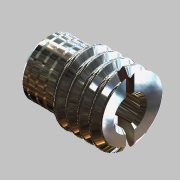
# Autodesk Inventor part: YTP-AP-E04-R1.0
Saved by Autodesk Inventor 2020.4 (Build 244396010, 396A)
## iProperties
Created: 2021-08-28
Part Number: YTP-AP-E04-R1.0
Material: Edelstahl
Document SubType Name: Modeling
Designer: Uwe Wieser
Mass: 0.28749 g
Surface Area: 1.23286 cm^2
Volume: 0.0359362 cm^3
Density: 8 g/cm^3
Appearance: Chrom - poliert
Project: Airbrush
Description: Dichtungsschraube
Werkstoff: 1.4301
Author: Uwe Wieser
Autodesk Inventor part; units mm, degrees
sketch "Skizze1" plane through (0, 0, 0) normal (0, 0, 1) x (1, 0, 0)
  line L0 (0, -0.4978) -> (0, 2.9869) projected
  line L1 (-3.8336, 0) -> (4.9014, 0) projected
  line L2 (-2.5857, 0.8) -> (-2.5857, 1.647)
  line L3 (2.4143, 2) -> (2.4143, 0.8)
  line L4 (-0.9352, 2) -> (-0.8754, 2) construction
  line L5 (-1.0857, 1.8366) -> (-0.8106, 1.8366) construction
  line L6 (-0.5857, 2) -> (-0.5857, 2.4891) construction
  line L7 (-1.5857, 2) -> (-1.5857, 2.1811) construction
  line L8 (-2.0857, 2) -> (-2.0857, 2.2584) construction
  line L9 (-2.0857, 1.4574) -> (-2.0167, 1.647)
  line L10 (-2.0857, 1.4574) -> (-2.1547, 1.647)
  line L11 (-0.5857, 2) -> (2.4143, 2)
  line L12 (-1.5166, 1.647) -> (-1.5876, 1.647) construction
  line L13 (-1.5166, 1.647) -> (-1.1547, 1.647)
  line L14 (-2.5857, 1.647) -> (-2.1547, 1.647)
  line L15 (-2.0167, 1.647) -> (-1.6548, 1.647)
  line L16 (-2.5857, 0.8) -> (2.4143, 0.8)
  line L17 (-1.1547, 1.647) -> (-1.0857, 1.4574)
  line L18 (-1.6548, 1.647) -> (-1.5856, 1.4574)
  line L19 (-1.5856, 1.4574) -> (-1.5166, 1.647)
  line L20 (-1.0857, 1.4574) -> (-1.0167, 1.647)
  line L21 (-1.0857, 1.4574) -> (-0.884, 1.4574) construction
  line L22 (-1.0167, 1.647) -> (-0.5857, 1.647)
  line L23 (-0.5857, 1.647) -> (-0.5857, 2)
  line L24 (3.2727, 1.57) -> (3.6536, 1.57) construction
  line L25 (2.4143, 1.8644) -> (3.0263, 1.8644) construction
  line L26 (2.4143, 1.8644) -> (3.0252, 1.8644) construction
  line L27 (3.3514, 1.57) -> (3.1921, 1.57) construction
  point P0 (0, 0)
  dimension "d7" = 2
  dimension "d8" = 0.5
  dimension "d9" = 0.5
  dimension "d10" = 0.5
  dimension "d16" = 1.6
  dimension "d19" = 3.294
  dimension "d21" = 70
  dimension "d22" = 4
  dimension "d42" = 5
  dimension "d43" = 110
  dimension "d44" = 110
  dimension "d45" = 0.1383
  dimension "d46" = 0.138
  dimension "d47" = 0.138
  dimension "d100" = 0.353
  constraints: 52 end point, 8 horizontal, 7 perpendicular, 3 horizontal alignment, 3 point on line, 3 symmetric about line, 3 vertical, 2 equal length
  measures "d7" distance from line of L6 L2.end
  measures "d8" distance from line of L6 L5.start
  measures "d9" distance from line of L5.start L7
  measures "d10" distance between parallel lines of L8 L7
  measures "d16" diameter of L16 L1
  measures "d19" diameter of L13 L1
  measures "d21" angle of L21 L20
  measures "d22" diameter of L11 L1
  measures "d42" distance of L3.end L2.start
  measures "d43" angle of L14 L10
  measures "d44" angle of L17 L13
  measures "d45" distance of L12.start L15.end
  measures "d46" distance of L9.end L10.end
  measures "d47" distance of L20.end L13.end
  measures "d100" distance of L22.end L6.start
revolve "Umdrehung1" add sketch "Skizze1" angle 360 about axis through (-10, 0, 0) along (1, 0, 0)
ref_plane "Arbeitsebene1" through (0, 0, 0) normal (0, 0, 1) x (1, 0, 0)
sketch "Skizze2" plane through (0, 0, 0) normal (0, 0, 1) x (1, 0, 0)
  line L0 (2.4143, -0.8) -> (2.4143, 0.8) projected
  line L1 (2.4143, -0.25) -> (1.4143, -0.25)
  line L2 (1.4143, -0.25) -> (1.4143, 0.25)
  line L3 (1.4143, 0.25) -> (2.4143, 0.25)
  line L4 (2.4143, 0.25) -> (2.4143, -0.25)
  line L5 (-0.4829, 0) -> (2.8972, 0) projected
  point P0 (0, 0)
  dimension "d52" = 1
  dimension "d53" = 0.5
  constraints: 8 end point, 2 parallel, 1 horizontal, 1 perpendicular, 1 point on line, 1 other
  measures "d52" distance of L3.end L2.end
  measures "d53" distance of L1.end L2.end
extrude "Extrusion1" cut sketch "Skizze2" along normal mid plane 10
chamfer "Fase1" distance 0.2 angle 45 3 edges at (2.4143, 0.6481, 0.469) (2.4143, 0.6481, -0.469) (2.4143, -0.8, 0)
ref_plane "Arbeitsebene2" through (0, 0, 0) normal (0, 1, 0) x (-1, 0, 0)
sketch "Skizze3" plane through (0, 0, 0) normal (0, 1, 0) x (-1, 0, 0)
  arc A0 (-2.4835, 2.001) -> (-2.5701, 1.951) centre (-2.4835, 1.901) ccw
  arc A1 (-3.0969, 1.951) -> (-3.1835, 2.001) centre (-3.1835, 1.901) ccw
  arc A2 (-2.9201, 1.6448) -> (-2.7469, 1.6448) centre (-2.8335, 1.6948) ccw
  line L0 (-3.1833, 1.571) -> (0.9975, 1.571) construction
  line L1 (-2.9201, 1.6448) -> (-3.0969, 1.951)
  line L2 (-2.7469, 1.6448) -> (-2.5701, 1.951)
  line L3 (-2.4835, 2.001) -> (-3.1835, 2.001) construction
  line L4 (0.5857, 2) -> (0.5857, -2) projected
  line L5 (-2.4835, 2.001) -> (-3.1835, 2.001)
  line L6 (-1.2513, 2) -> (-2.6585, 2) construction
  point P0 (0, 0)
  dimension "d67" = 0.2
  dimension "d68" = 0.2
  dimension "d69" = 0.2
  dimension "d70" = 60
  dimension "d71" = 60
  dimension "d72" = 0.43
  dimension "d123" = 0.7
  constraints: 12 end point, 7 point on circle, 6 tangent, 3 centre point, 3 horizontal, 1 horizontal alignment, 1 point on line
  measures "d67" diameter of A0
  measures "d68" diameter of A1
  measures "d69" diameter of A2
  measures "d70" angle of L1 L2
  measures "d71" angle of L0 L1
  measures "d72" distance between parallel lines of L3 L0
  measures "d123" distance of L3.end point (-2.483, 2.001)
chamfer "Fase2" distance 0.2 angle 45 1 edges at (-2.5857, -1.647, 0)
sketch "Skizze4" plane through (0, 0, 0) normal (0, 1, 0) x (-1, 0, 0)
  point P0 (0, 0)
chamfer "Fase3" distance 0.25 angle 45 1 edges at (-0.5857, -2, 0)
ref_plane "Arbeitsebene3" through (-0.6, 0, 0) normal (1, 0, 0) x (0, 1, 0)
sketch "Skizze5" plane through (-0.6, 0, 0) normal (1, 0, 0) x (0, 1, 0)
  circle A0 centre (0, 0) radius 1.6479
  circle A1 centre (0, 0) radius 0.8
  dimension "d105" = 1.6
  constraints: 2 centre point, 2 coincident
  measures "d105" diameter of A1
extrude "Extrusion2" add sketch "Skizze5" against normal blind 2
sketch "Skizze6" plane through (0, 0, 0) normal (0, 1, 0) x (-1, 0, 0)
  line L0 (1.1, 1.4583) -> (1.169, 1.6479)
  line L1 (1.1, 1.4583) -> (1.031, 1.6479)
  line L2 (1.6691, 1.6479) -> (1.5981, 1.6479) construction
  line L3 (2.031, 1.6479) -> (2.1, 1.4583)
  line L4 (1.5309, 1.6479) -> (1.6001, 1.4583)
  line L5 (1.6001, 1.4583) -> (1.6691, 1.6479)
  line L6 (2.1, 1.4583) -> (2.169, 1.6479)
  line L7 (2.1, 1.4583) -> (2.3017, 1.4583) construction
  line L8 (2.169, 1.6479) -> (2.031, 1.6479)
  line L9 (1.6691, 1.6479) -> (1.5309, 1.6479)
  line L10 (1.169, 1.6479) -> (1.031, 1.6479)
  line L11 (2.6, -1.6479) -> (2.6, 1.6479) projected
  line L12 (3.6403, 0) -> (-3.6419, 0) projected
  point P0 (0, 0)
  dimension "d108" = 70
  dimension "d111" = 0.1383
  dimension "d112" = 0.138
  dimension "d113" = 0.138
  dimension "d114" = 0.5
  dimension "d115" = 0.4999
  dimension "d116" = 0.5001
  dimension "d117" = 0.1896
  dimension "d118" = 1.4583
  constraints: 22 end point, 3 horizontal, 3 horizontal alignment, 2 collinear, 2 equal length
  measures "d108" angle of L7 L6
  measures "d111" distance of L5.end L4.start
  measures "d112" distance of L0.end L1.end
  measures "d113" distance of L6.end L3.start
  measures "d114" distance from line of L11 L7.start
  measures "d115" distance of L5.start L7.start
  measures "d116" distance of L0.start L5.start
  measures "d117" vertical distance of L7.start L6.end
  measures "d118" distance from line of L12 L0.start
revolve "Umdrehung2" cut sketch "Skizze6" angle 360 about axis through (-10, 0, 0) along (1, 0, 0)
chamfer "Fase4" distance 0.2 angle 45 1 edges at (-2.6, -1.6479, 0)
coil "Spirale4" sketch "Skizze3" operation cut axis through (-10, 0, 0) along (-1, 0, 0) pitch 0.7 turns 5.714286 hand right
